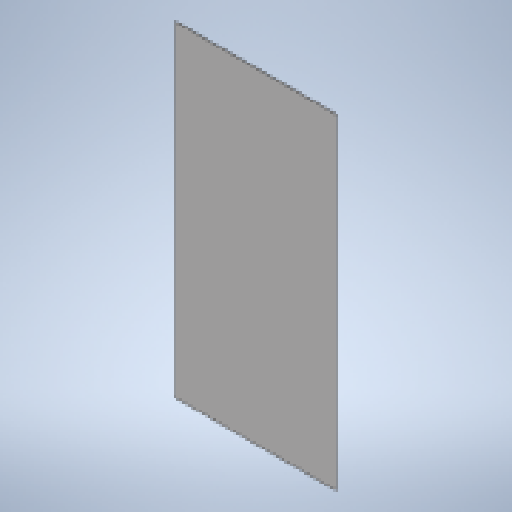
# Autodesk Inventor part: GBK 2231 shield 6
Saved by Autodesk Inventor 2026.2 (Build 302298000, 298)
## iProperties
Created: 2026-04-17
Part Number: GBK 2231 shield 6
Material: Steel
Document SubType Name: Sheet Metal
Designer: pokla
Stock Number: 2236
Mass: 138487 g
Surface Area: 88564.8 cm^2
Volume: 17641.6 cm^3
Density: 7.85 g/cm^3
Flat Pattern Width: 148 cm
Flat Pattern Length: 285.636 cm
Flat Pattern Area: 42274.1 cm^2
Sheet Metal Rule: Default_mm
Sheet Metal Width: 1480,000 mm
Sheet Metal Length: 2856,360 mm
Sheet Metal Area: 4227412,869 mm^2
Appearance: Default
Author: admin
Autodesk Inventor part; units mm, degrees
ref_plane "YZ Plane" through (0, 0, 0) normal (1, 0, 0) x (0, 1, 0)
ref_plane "XZ Plane" through (0, 0, 0) normal (0, 1, 0) x (-1, 0, 0)
ref_plane "XY Plane" through (0, 0, 0) normal (0, 0, 1) x (1, 0, 0)
sketch "Sketch1" plane through (0, 0, 0) normal (0, 0, 1) x (1, 0, 0)
  line L0 (740, -1490) -> (-740, -1490)
  line L1 (-740, -1490) -> (-740, 1490)
  line L2 (-740, 1490) -> (740, 1490)
  line L3 (740, 1490) -> (740, -1490)
  line L4 (740, -1490) -> (-740, 1490) construction
  line L5 (-740, -1490) -> (740, 1490) construction
  line L6 (740, 1366.36) -> (-740, 1332.7741)
  point P0 (0, 0)
  dimension "d0" = 1480
  dimension "d1" = 2980
  dimension "d3" = 1.3
  measures "d0" distance of L1.end L2.end
  measures "d1" distance of L0.end L1.end
  measures "d3" angle of L2 L6
extrude "Plate1" add sketch "Sketch1" along normal blind 4 contours L0 L1 L6 L3
sketch "Sketch2" plane through (0, 0, 4) normal (0, 0, 1) x (1, 0, 0)
  line L0 (455.1539, 1018.8602) -> (455.1539, 661.1698) construction
  line L1 (455.1539, 661.1698) -> (423.8897, 661.1698) construction
  line L2 (423.8897, 661.1698) -> (423.8897, 1018.8602) construction
  line L3 (423.8897, 1018.8602) -> (455.1539, 1018.8602) construction
  point P0 (0, 0)
  constraints: 2 other
equation "\"d0\" = Лист_ширина"
equation "\"d2\" = Thickness"
equation "\"BendRadius\" = Thickness"
equation "\"BendReliefWidth\" = Thickness"
equation "\"BendReliefDepth\" = 0.5 * Thickness"
equation "\"CornerReliefSize\" = 4 * Thickness"
equation "\"MinimumRemnant\" = 2 * Thickness"
equation "\"TransitionRadius\" = BendRadius"
equation "\"JacobiRadiusSize\" = BendRadius"
equation "\"GapSize\" = Thickness"
equation "\"Лист_ширина\" = 1480"
equation "\"Thickness\" = 4"
body "Solid1"
